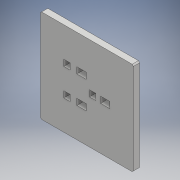
# Autodesk Inventor part: Socle_Testbench
Saved by Autodesk Inventor 2017 (Build 210142000, 142)
## iProperties
Part Number: Socle_Testbench
Material: Générique
Document SubType Name: Modeling
Designer: Darren
Density: 1 g/cm^3
Appearance: Par défaut
Author: Darren
Autodesk Inventor part; units mm, degrees
ref_plane "YZ Plane" through (0, 0, 0) normal (1, 0, 0) x (0, 1, 0)
ref_plane "XZ Plane" through (0, 0, 0) normal (0, 1, 0) x (-1, 0, 0)
ref_plane "XY Plane" through (0, 0, 0) normal (0, 0, 1) x (1, 0, 0)
sketch "Esquisse4" plane through (0, 0, 0) normal (0, 1, 0) x (-1, 0, 0)
  line L0 (37.83, -34.9448) -> (22.83, -34.9448) construction
  line L1 (37.83, -34.9448) -> (37.83, -24.9448) construction
  line L2 (22.83, -24.9448) -> (37.83, -24.9448) construction
  line L3 (22.83, -34.9448) -> (22.83, -24.9448) construction
  line L4 (55.83, -34.9448) -> (45.83, -34.9448) construction
  line L5 (55.83, -34.9448) -> (55.83, -24.9448) construction
  line L6 (45.83, -24.9448) -> (55.83, -24.9448) construction
  line L7 (45.83, -34.9448) -> (45.83, -24.9448) construction
  line L8 (76.13, -13.0448) -> (61.13, -13.0448) construction
  line L9 (76.13, -13.0448) -> (76.13, -3.0448) construction
  line L10 (61.13, -3.0448) -> (76.13, -3.0448) construction
  line L11 (61.13, -13.0448) -> (61.13, -3.0448) construction
  line L12 (97.13, -13.0448) -> (87.13, -13.0448) construction
  line L13 (97.13, -13.0448) -> (97.13, -3.0448) construction
  line L14 (87.13, -3.0448) -> (97.13, -3.0448) construction
  line L15 (87.13, -13.0448) -> (87.13, -3.0448) construction
  line L16 (76.13, -57.0448) -> (61.13, -57.0448) construction
  line L17 (76.13, -57.0448) -> (76.13, -47.0448) construction
  line L18 (61.13, -47.0448) -> (76.13, -47.0448) construction
  line L19 (61.13, -57.0448) -> (61.13, -47.0448) construction
  line L20 (97.13, -57.0448) -> (87.13, -57.0448) construction
  line L21 (97.13, -57.0448) -> (97.13, -47.0448) construction
  line L22 (87.13, -47.0448) -> (97.13, -47.0448) construction
  line L23 (87.13, -57.0448) -> (87.13, -47.0448) construction
  line L24 (-13.02, 45.0552) -> (132.98, 45.0552)
  line L25 (134.98, 43.0552) -> (134.98, -102.9448)
  line L26 (132.98, -104.9448) -> (-13.02, -104.9448)
  line L27 (-15.02, -102.9448) -> (-15.02, 43.0552)
  line L28 (22.83, -24.9448) -> (37.83, -24.9448)
  line L29 (37.83, -24.9448) -> (37.83, -34.9448)
  line L30 (37.83, -34.9448) -> (22.83, -34.9448)
  line L31 (22.83, -34.9448) -> (22.83, -24.9448)
  line L32 (45.83, -24.9448) -> (55.83, -24.9448)
  line L33 (55.83, -24.9448) -> (55.83, -34.9448)
  line L34 (55.83, -34.9448) -> (45.83, -34.9448)
  line L35 (45.83, -34.9448) -> (45.83, -24.9448)
  line L36 (61.13, -3.0448) -> (76.13, -3.0448)
  line L37 (76.13, -3.0448) -> (76.13, -13.0448)
  line L38 (76.13, -13.0448) -> (61.13, -13.0448)
  line L39 (61.13, -13.0448) -> (61.13, -3.0448)
  line L40 (87.13, -3.0448) -> (97.13, -3.0448)
  line L41 (97.13, -3.0448) -> (97.13, -13.0448)
  line L42 (97.13, -13.0448) -> (87.13, -13.0448)
  line L43 (87.13, -13.0448) -> (87.13, -3.0448)
  line L44 (61.13, -47.0448) -> (76.13, -47.0448)
  line L45 (76.13, -47.0448) -> (76.13, -57.0448)
  line L46 (76.13, -57.0448) -> (61.13, -57.0448)
  line L47 (61.13, -57.0448) -> (61.13, -47.0448)
  line L48 (87.13, -47.0448) -> (97.13, -47.0448)
  line L49 (97.13, -47.0448) -> (97.13, -57.0448)
  line L50 (97.13, -57.0448) -> (87.13, -57.0448)
  line L51 (87.13, -57.0448) -> (87.13, -47.0448)
  line L52 (132.98, 45.0552) -> (134.98, 43.0552)
  line L53 (-13.02, 45.0552) -> (-15.02, 43.0552)
  line L54 (-15.02, -102.9448) -> (-13.02, -104.9448)
  line L55 (132.98, -104.9448) -> (134.98, -102.9448)
  line L56 (45.83, -29.9448) -> (55.83, -29.9448) construction
  line L57 (97.13, -3.0448) -> (22.83, -3.0448) construction
  line L58 (22.83, -3.0448) -> (22.83, -57.0448) construction
  line L59 (22.83, -57.0448) -> (97.13, -57.0448) construction
  line L60 (97.13, -57.0448) -> (97.13, -3.0448) construction
  line L61 (22.83, -3.0448) -> (59.98, -3.0448) construction
  line L62 (59.98, -3.0448) -> (59.98, -57.0448) construction
  point P0 (0, 0)
  point P1 (-15.02, 45.0552)
  point P2 (134.98, -104.9448)
  point P3 (134.98, 45.0552)
  point P4 (-15.02, -104.9448)
  dimension "d20" = 150
  dimension "d21" = 150
  dimension "d26" = 2
  dimension "d27" = 2
  dimension "d28" = 2
  dimension "d29" = 2
  dimension "d30" = 2
  dimension "d31" = 2
  dimension "d32" = 2
  dimension "d33" = 2
  dimension "d34" = 37.15
  dimension "d35" = 75
  dimension "d36" = 75
  constraints: 78 end point, 16 parallel, 8 horizontal, 8 perpendicular, 8 point on line, 4 midpoint
  measures "d20" distance of point (134.98, -104.945) point (-15.02, -104.945)
  measures "d21" distance of point (134.98, 45.055) point (134.98, -104.945)
  measures "d26" distance of L24.end point (134.98, 45.055)
  measures "d27" distance of L25.start point (134.98, 45.055)
  measures "d28" distance of L24.start point (-15.02, 45.055)
  measures "d29" distance of L27.end point (-15.02, 45.055)
  measures "d30" distance of L27.start point (-15.02, -104.945)
  measures "d31" distance of L26.end point (-15.02, -104.945)
  measures "d32" distance of L26.start point (134.98, -104.945)
  measures "d33" distance of L25.end point (134.98, -104.945)
  measures "d34" distance of L57.end L61.end
  measures "d35" distance between parallel lines of L27 L62
  measures "d36" distance between parallel lines of L56 L24
extrude "Extrusion4" add sketch "Esquisse4" along normal blind 10
equation "\"d27\" = d26"
equation "\"d28\" = d26"
equation "\"d29\" = d28"
equation "\"d30\" = d26"
equation "\"d31\" = d30"
equation "\"d32\" = d26"
equation "\"d33\" = d32"
